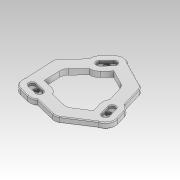
# Autodesk Inventor part: ValveThing2
Saved by Autodesk Inventor 2020 (Build 240168000, 168)
## iProperties
Created: 2022-01-09
Part Number: ValveThing2
Material: Generic
Document SubType Name: Modeling
Designer: DDeGo
Density: 1 g/cm^3
Appearance: Default
Author: DDeGo
Autodesk Inventor part; units mm, degrees
ref_plane "YZ Plane" through (0, 0, 0) normal (1, 0, 0) x (0, 1, 0)
ref_plane "XZ Plane" through (0, 0, 0) normal (0, 1, 0) x (-1, 0, 0)
ref_plane "XY Plane" through (0, 0, 0) normal (0, 0, 1) x (1, 0, 0)
sketch "Block1" plane through (0, 0, 0) normal (0, 0, 1) x (1, 0, 0)
  circle A0 centre (-3.875, 6.7117) radius 2.6
  arc A1 (-0.9902, 6.6954) -> (-5.6639, 8.975) centre (-3.327, 7.8352) ccw
  line L0 (-0.9902, 6.6954) -> (-1.5381, 5.5719)
  line L1 (-6.2119, 7.8515) -> (-5.6639, 8.975)
  line L2 (-1.5381, 5.5719) -> (-2.0861, 4.4484)
  arc A2 (-1.5381, 5.5719) -> (-6.2119, 7.8515) centre (-3.875, 6.7117) ccw
  circle A3 centre (-3.875, 6.7117) radius 1.25
  line L3 (-6.7598, 6.728) -> (-6.2119, 7.8515)
  arc A4 (-6.2119, 7.8515) -> (-1.5381, 5.5719) centre (-3.875, 6.7117) ccw
  arc A5 (-6.7598, 6.728) -> (-2.0861, 4.4484) centre (-4.423, 5.5882) ccw
  line L4 (4.6199, 1.9581) -> (1.25, 6.9542)
  line L5 (1.8, 11.5037) -> (7.107, 3.6357)
  line L6 (-5.3033, -4.2052) -> (-4.0564, -4.118)
  line L7 (-3.6936, -9.3054) -> (-4.9406, -9.3926)
  arc A6 (-4.0564, -4.118) -> (-3.6936, -9.3054) centre (-3.875, -6.7117) ccw
  line L8 (-4.0564, -4.118) -> (-2.8094, -4.0308)
  circle A7 centre (-3.875, -6.7117) radius 1.25
  circle A8 centre (-3.875, -6.7117) radius 2.6
  line L9 (-2.4467, -9.2182) -> (-3.6936, -9.3054)
  arc A9 (-3.6936, -9.3054) -> (-4.0564, -4.118) centre (-3.875, -6.7117) ccw
  arc A10 (-2.4467, -9.2182) -> (-2.8094, -4.0308) centre (-2.628, -6.6245) ccw
  arc A11 (-0.4049, -7.9727) -> (-0.6142, -4.98) centre (-2.628, -6.6245) ccw
  arc A12 (-6.6475, -2.3946) -> (-6.4003, -4.5348) centre (-4.8499, -3.2713) ccw
  line L10 (-4.0057, 3.0219) -> (-6.6475, -2.3946)
  line L11 (-10.8625, -4.193) -> (-6.7021, 4.337)
  arc A13 (-6.7021, 4.337) -> (-4.0057, 3.0219) centre (-4.423, 5.5882) ccw
  arc A14 (9.2065, 2.4902) -> (4.8955, -0.4176) centre (7.051, 1.0363) ccw
  line L12 (5.5945, -1.4539) -> (4.8955, -0.4176)
  line L13 (9.2065, 2.4902) -> (9.9055, 1.4539)
  circle A15 centre (7.75, 0) radius 1.25
  line L14 (9.9055, 1.4539) -> (10.6045, 0.4176)
  arc A16 (9.9055, 1.4539) -> (5.5945, -1.4539) centre (7.75, 0) ccw
  circle A17 centre (7.75, 0) radius 2.6
  arc A18 (5.5945, -1.4539) -> (9.9055, 1.4539) centre (7.75, 0) ccw
  arc A19 (6.2935, -2.4902) -> (10.6045, 0.4176) centre (8.449, -1.0363) ccw
  arc A20 (7.1274, -3.2754) -> (10.8801, -1.9581) centre (8.449, -1.0363) ccw
  line L15 (10.8801, -1.9581) -> (11.3403, -2.6404)
  arc A21 (7.107, 3.6357) -> (4.6199, 1.9581) centre (7.051, 1.0363) ccw
  arc A22 (9.0625, -7.3107) -> (11.3403, -2.6404) centre (8.8532, -4.318) ccw
  arc A23 (5.3975, -4.5596) -> (7.1274, -3.2754) centre (5.258, -2.5645) ccw
  line L16 (9.0625, -7.3107) -> (-0.4049, -7.9727)
  line L17 (-0.6142, -4.98) -> (5.3975, -4.5596)
  line L18 (6.2935, -2.4902) -> (5.5945, -1.4539)
  arc A24 (-5.3033, -4.2052) -> (-4.9406, -9.3926) centre (-5.122, -6.7989) ccw
  arc A25 (-6.4003, -4.5348) -> (-7.1358, -8.4434) centre (-5.122, -6.7989) ccw
  line L19 (-7.1358, -8.4434) -> (-7.9568, -8.5008)
  arc A26 (-10.8625, -4.193) -> (-7.9568, -8.5008) centre (-8.1661, -5.5081) ccw
  arc A27 (-0.7272, 7.8102) -> (-3.7443, 10.4015) centre (-3.327, 7.8352) ccw
  line L20 (-3.7443, 10.4015) -> (-3.3835, 11.1412)
  arc A28 (1.25, 6.9542) -> (-0.7272, 7.8102) centre (-0.4081, 5.8358) ccw
  arc A29 (1.8, 11.5037) -> (-3.3835, 11.1412) centre (-0.6871, 9.8261) ccw
  point P0 (0, 0)
sketch "Block2" plane through (0, 0, 0) normal (0, 0, 1) x (1, 0, 0)
  line L0 (-0.9902, 6.6954) -> (-2.0861, 4.4484)
  arc A0 (-4.0057, 3.0219) -> (-2.0861, 4.4484) centre (-4.423, 5.5882) ccw
  arc A1 (-6.7598, 6.728) -> (-6.7021, 4.337) centre (-4.423, 5.5882) ccw
  circle A2 centre (-3.875, 6.7117) radius 2.1
  line L1 (-6.7598, 6.728) -> (-5.6639, 8.975)
  arc A3 (-2.1873, 10.1721) -> (-5.6639, 8.975) centre (-3.327, 7.8352) ccw
  arc A4 (-0.9902, 6.6954) -> (-0.9193, 6.8539) centre (-3.327, 7.8352) ccw
  line L2 (0.8695, 6.4912) -> (-0.9193, 6.8539)
  line L3 (-2.1873, 10.1721) -> (2.6696, 9.1872)
  arc A5 (2.1301, 5.6494) -> (0.8695, 6.4912) centre (0.472, 4.5311) ccw
  arc A6 (3.9302, 8.3455) -> (2.6696, 9.1872) centre (2.2722, 7.2271) ccw
  line L4 (3.9302, 8.3455) -> (7.107, 3.6357)
  line L5 (4.6199, 1.9581) -> (2.1301, 5.6494)
  line L6 (-0.6142, -4.98) -> (3.8275, -4.6694)
  line L7 (5.2623, -7.5764) -> (-0.4049, -7.9727)
  arc A7 (5.2623, -7.5764) -> (6.6215, -6.9056) centre (5.1228, -5.5813) ccw
  line L8 (9.9029, -3.1918) -> (6.6215, -6.9056)
  arc A8 (9.9029, -3.1918) -> (10.6045, 0.4176) centre (8.449, -1.0363) ccw
  line L9 (9.2065, 2.4902) -> (10.6045, 0.4176)
  arc A9 (9.2065, 2.4902) -> (7.107, 3.6357) centre (7.051, 1.0363) ccw
  arc A10 (4.6199, 1.9581) -> (4.8955, -0.4176) centre (7.051, 1.0363) ccw
  line L10 (6.2935, -2.4902) -> (4.8955, -0.4176)
  arc A11 (6.2935, -2.4902) -> (6.3953, -2.6308) centre (8.449, -1.0363) ccw
  arc A12 (3.8275, -4.6694) -> (5.1868, -3.9986) centre (3.688, -2.6743) ccw
  line L11 (5.1868, -3.9986) -> (6.3953, -2.6308)
  circle A13 centre (7.75, 0) radius 2.1
  line L12 (-7.7156, -6.9803) -> (-9.2912, -2.2816)
  arc A14 (-7.7156, -6.9803) -> (-4.9406, -9.3926) centre (-5.122, -6.7989) ccw
  line L13 (-2.4467, -9.2182) -> (-4.9406, -9.3926)
  arc A15 (-2.4467, -9.2182) -> (-0.4049, -7.9727) centre (-2.628, -6.6245) ccw
  line L14 (-5.3033, -4.2052) -> (-2.8094, -4.0308)
  arc A16 (-5.3033, -4.2052) -> (-5.476, -4.2231) centre (-5.122, -6.7989) ccw
  circle A17 centre (-3.875, -6.7117) radius 2.1
  arc A18 (-0.6142, -4.98) -> (-2.8094, -4.0308) centre (-2.628, -6.6245) ccw
  line L15 (-4.0057, 3.0219) -> (-5.9576, -0.98)
  line L16 (-9.1925, -0.7691) -> (-6.7021, 4.337)
  arc A19 (-5.9576, -0.98) -> (-6.0562, -2.4926) centre (-4.16, -1.8568) ccw
  line L17 (-6.0562, -2.4926) -> (-5.476, -4.2231)
  arc A20 (-9.1925, -0.7691) -> (-9.2912, -2.2816) centre (-7.3949, -1.6458) ccw
  point P0 (0, 0)
  point P1 (0, 0)
sketch "Sketch6" plane through (0, 0, 0) normal (0, 1, 0) x (-1, 0, 0)
  arc A0 (-45, -21.7945) -> (-45, 21.7945) centre (0, 0) ccw
  line L0 (-45, 21.7945) -> (-45, -21.7945)
  dimension "d22" = 50
  dimension "d23" = 45
  constraints: 2 end point, 2 point on circle, 1 centre point, 1 coincident, 1 vertical
  measures "d22" radius of A0
  measures "d23" distance from line of L0 point (0, 0)
extrude "Extrusion6" add sketch "Sketch6" along normal blind 1.4
sketch "Sketch7" plane through (0, 1.4, 0) normal (0, 1, 0) x (1, 0, 0)
  arc A0 (7.5335, 6.4999) -> (6.53, 7.7139) centre (5.6147, 5.9356) ccw projected
  line L0 (0.2576, 10.9422) -> (6.53, 7.7139) projected
  arc A1 (0.2576, 10.9422) -> (-3.4183, 10.8532) centre (-1.5358, 9.0597) ccw projected
  line L1 (-5.1427, 9.0431) -> (-3.4183, 10.8532) projected
  arc A2 (-5.1427, 9.0431) -> (-5.8481, 6.998) centre (-3.2603, 7.2497) ccw projected
  line L2 (-9.3958, 3.2742) -> (-5.8481, 6.998) projected
  arc A3 (-9.3958, 3.2742) -> (-9.9454, 1.7981) centre (-7.9478, 1.8947) ccw projected
  line L3 (-9.605, -5.248) -> (-9.9454, 1.7981) projected
  arc A4 (-9.605, -5.248) -> (-7.69, -8.3869) centre (-7.078, -5.8599) ccw projected
  line L4 (-5.2602, -8.9753) -> (-7.69, -8.3869) projected
  arc A5 (-5.2602, -8.9753) -> (-3.1364, -8.5636) centre (-4.6483, -6.4483) ccw projected
  line L5 (1.8623, -9.7741) -> (-3.1364, -8.5636) projected
  arc A6 (1.8623, -9.7741) -> (3.4155, -9.5121) centre (2.3331, -7.8303) ccw projected
  line L6 (9.3474, -5.6942) -> (3.4155, -9.5121) projected
  arc A7 (9.3474, -5.6942) -> (11.1083, -2.4663) centre (8.6139, -3.1998) ccw projected
  line L7 (10.4029, -0.0678) -> (11.1083, -2.4663) projected
  arc A8 (10.4029, -0.0678) -> (8.9845, 1.5656) centre (7.9086, -0.8013) ccw projected
  line L8 (7.5335, 6.4999) -> (8.9845, 1.5656) projected
  arc A9 (5.7226, 0.6064) -> (5.4142, -1.5349) centre (7.9086, -0.8013) ccw projected
  line L9 (6.0688, -3.761) -> (5.4142, -1.5349) projected
  line L10 (2.8001, -5.8648) -> (6.0688, -3.761) projected
  arc A10 (1.247, -6.1268) -> (2.8001, -5.8648) centre (1.7177, -4.183) ccw projected
  line L11 (-2.3362, -5.2591) -> (1.247, -6.1268) projected
  arc A11 (-2.3362, -5.2591) -> (-4.0363, -3.9214) centre (-4.6483, -6.4483) ccw projected
  line L12 (-6.2915, -3.3753) -> (-4.0363, -3.9214) projected
  line L13 (-6.4791, 0.5074) -> (-6.2915, -3.3753) projected
  arc A12 (-5.9295, 1.9835) -> (-6.4791, 0.5074) centre (-4.4814, 0.6039) ccw projected
  line L14 (-3.3864, 4.6527) -> (-5.9295, 1.9835) projected
  arc A13 (-3.3864, 4.6527) -> (-1.3779, 5.4563) centre (-3.2603, 7.2497) ccw projected
  line L15 (0.2227, 7.1362) -> (-1.3779, 5.4563) projected
  line L16 (3.679, 5.3574) -> (0.2227, 7.1362) projected
  arc A14 (4.6825, 4.1433) -> (3.679, 5.3574) centre (2.7637, 3.5791) ccw projected
  line L17 (5.7226, 0.6064) -> (4.6825, 4.1433) projected
  circle A15 centre (-5.8632, -6.1541) radius 2.1 projected
  circle A16 centre (-2.3981, 8.1547) radius 2.1 projected
  circle A17 centre (8.2612, -2.0006) radius 2.1 projected
  line L18 (45, -21.7945) -> (45, 21.7945) projected
  arc A18 (45, 21.7945) -> (45, -21.7945) centre (0, 0) ccw projected
extrude "Extrusion7" cut sketch "Sketch7" against normal through all contours A9 L9 L10 A10 L11 A11 L12 L13 A12 L14 A13 L15 L16 A14 L17 | A18 L18
sketch "Sketch8" plane through (0, 1.4, 0) normal (0, 1, 0) x (1, 0, 0)
  line L0 (4.6825, 4.1433) -> (5.7226, 0.6064) projected
  arc A0 (5.7226, 0.6064) -> (5.4142, -1.5349) centre (7.9086, -0.8013) ccw projected
  line L1 (5.4142, -1.5349) -> (6.0688, -3.761) projected
  line L2 (6.0688, -3.761) -> (2.8001, -5.8648) projected
  arc A1 (1.247, -6.1268) -> (2.8001, -5.8648) centre (1.7177, -4.183) ccw projected
  line L3 (1.247, -6.1268) -> (-2.3362, -5.2591) projected
  arc A2 (-2.3362, -5.2591) -> (-4.0363, -3.9214) centre (-4.6483, -6.4483) ccw projected
  line L4 (-4.0363, -3.9214) -> (-6.2915, -3.3753) projected
  line L5 (-6.2915, -3.3753) -> (-6.4791, 0.5074) projected
  arc A3 (-5.9295, 1.9835) -> (-6.4791, 0.5074) centre (-4.4814, 0.6039) ccw projected
  line L6 (-5.9295, 1.9835) -> (-3.3864, 4.6527) projected
  arc A4 (-3.3864, 4.6527) -> (-1.3779, 5.4563) centre (-3.2603, 7.2497) ccw projected
  line L7 (-1.3779, 5.4563) -> (0.2227, 7.1362) projected
  line L8 (0.2227, 7.1362) -> (3.679, 5.3574) projected
  arc A5 (4.6825, 4.1433) -> (3.679, 5.3574) centre (2.7637, 3.5791) ccw projected
  line L9 (-3.4183, 10.8532) -> (-5.1427, 9.0431) projected
  arc A6 (-5.1427, 9.0431) -> (-5.8481, 6.998) centre (-3.2603, 7.2497) ccw projected
  line L10 (-5.8481, 6.998) -> (-9.3958, 3.2742) projected
  arc A7 (-9.3958, 3.2742) -> (-9.9454, 1.7981) centre (-7.9478, 1.8947) ccw projected
  line L11 (-9.9454, 1.7981) -> (-9.605, -5.248) projected
  arc A8 (-9.605, -5.248) -> (-7.69, -8.3869) centre (-7.078, -5.8599) ccw projected
  line L12 (-7.69, -8.3869) -> (-5.2602, -8.9753) projected
  arc A9 (-5.2602, -8.9753) -> (-3.1364, -8.5636) centre (-4.6483, -6.4483) ccw projected
  line L13 (-3.1364, -8.5636) -> (1.8623, -9.7741) projected
  arc A10 (1.8623, -9.7741) -> (3.4155, -9.5121) centre (2.3331, -7.8303) ccw projected
  line L14 (3.4155, -9.5121) -> (9.3474, -5.6942) projected
  arc A11 (9.3474, -5.6942) -> (11.1083, -2.4663) centre (8.6139, -3.1998) ccw projected
  line L15 (11.1083, -2.4663) -> (10.4029, -0.0678) projected
  arc A12 (10.4029, -0.0678) -> (8.9845, 1.5656) centre (7.9086, -0.8013) ccw projected
  line L16 (8.9845, 1.5656) -> (7.5335, 6.4999) projected
  arc A13 (7.5335, 6.4999) -> (6.53, 7.7139) centre (5.6147, 5.9356) ccw projected
  line L17 (6.53, 7.7139) -> (0.2576, 10.9422) projected
  arc A14 (0.2576, 10.9422) -> (-3.4183, 10.8532) centre (-1.5358, 9.0597) ccw projected
  arc A15 (-5.0341, 8.9397) -> (-5.6913, 6.9451) centre (-3.2603, 7.2497) ccw
  line L18 (-5.0341, 8.9397) -> (-3.3097, 10.7497)
  arc A16 (0.1695, 10.8188) -> (-3.3097, 10.7497) centre (-1.5358, 9.0597) ccw
  line L19 (0.1695, 10.8188) -> (6.4613, 7.5806)
  arc A17 (7.3896, 6.4576) -> (6.4613, 7.5806) centre (5.6147, 5.9356) ccw
  line L20 (7.3896, 6.4576) -> (8.8603, 1.4562)
  arc A18 (10.259, -0.1101) -> (8.8603, 1.4562) centre (7.9086, -0.8013) ccw
  line L21 (10.259, -0.1101) -> (10.9643, -2.5086)
  arc A19 (9.2846, -5.5562) -> (10.9643, -2.5086) centre (8.6139, -3.1998) ccw
  line L22 (9.2846, -5.5562) -> (3.3343, -9.3859)
  arc A20 (1.8976, -9.6283) -> (3.3343, -9.3859) centre (2.3331, -7.8303) ccw
  line L23 (1.8976, -9.6283) -> (-3.169, -8.4014)
  arc A21 (-5.2249, -8.8295) -> (-3.169, -8.4014) centre (-4.6483, -6.4483) ccw
  line L24 (-5.2249, -8.8295) -> (-7.6547, -8.2411)
  arc A22 (-9.4541, -5.2627) -> (-7.6547, -8.2411) centre (-7.078, -5.8599) ccw
  line L25 (-9.4541, -5.2627) -> (-9.7956, 1.8054)
  arc A23 (-9.2872, 3.1708) -> (-9.7956, 1.8054) centre (-7.9478, 1.8947) ccw
  line L26 (-9.2872, 3.1708) -> (-5.6913, 6.9451)
  line L27 (2.8813, -5.9909) -> (6.2444, -3.8264)
  line L28 (6.2444, -3.8264) -> (5.5581, -1.4926)
  arc A24 (5.8862, 0.5816) -> (5.5581, -1.4926) centre (7.9086, -0.8013) ccw
  line L29 (5.8862, 0.5816) -> (4.8264, 4.1856)
  arc A25 (4.8264, 4.1856) -> (3.7476, 5.4907) centre (2.7637, 3.5791) ccw
  line L30 (3.7476, 5.4907) -> (0.1915, 7.321)
  line L31 (0.1915, 7.321) -> (-1.4865, 5.5597)
  arc A26 (-3.4468, 4.8068) -> (-1.4865, 5.5597) centre (-3.2603, 7.2497) ccw
  line L32 (-3.4468, 4.8068) -> (-6.0381, 2.087)
  arc A27 (-6.0381, 2.087) -> (-6.6289, 0.5002) centre (-4.4814, 0.6039) ccw
  line L33 (-6.6289, 0.5002) -> (-6.4359, -3.4946)
  line L34 (-6.4359, -3.4946) -> (-4.0716, -4.0672)
  arc A28 (-2.4394, -5.3885) -> (-4.0716, -4.0672) centre (-4.6483, -6.4483) ccw
  line L35 (-2.4394, -5.3885) -> (1.2117, -6.2726)
  arc A29 (1.2117, -6.2726) -> (2.8813, -5.9909) centre (1.7177, -4.183) ccw
  point P0 (0, 0)
  dimension "d28" = 0.15
  dimension "d33" = 0.15
  constraints: 36 end point, 30 point on circle, 15 centre point, 31 other
  measures "d28" distance between parallel lines of L10 L26
  measures "d33" distance between parallel lines of L6 L32
extrude "Extrusion8" cut sketch "Sketch8" against normal through all
sketch "Sketch2" plane through (0, 1.4, 1.4) normal (0, 1, 0) x (1, 0, 0)
  line L0 (-4.6483, -5.0483) -> (-7.078, -4.4599) construction
  line L1 (-4.813, -5.7287) -> (-7.2428, -5.1403)
  line L2 (-6.9133, -3.7796) -> (-4.4835, -4.368)
  arc A0 (-4.813, -5.7287) -> (-4.4835, -4.368) centre (-4.6483, -5.0483) ccw
  arc A1 (-6.9133, -3.7796) -> (-7.2428, -5.1403) centre (-7.078, -4.4599) ccw
  line L3 (7.9086, 0.5987) -> (8.6139, -1.7998) construction
  line L4 (7.237, 0.4012) -> (7.9423, -1.9973)
  line L5 (9.2854, -1.6023) -> (8.5801, 0.7961)
  arc A2 (8.5801, 0.7961) -> (7.237, 0.4012) centre (7.9086, 0.5987) ccw
  arc A3 (7.9423, -1.9973) -> (9.2854, -1.6023) centre (8.6139, -1.7998) ccw
  line L6 (-3.2603, 8.6497) -> (-1.5358, 10.4597) construction
  line L7 (-3.7671, 9.1325) -> (-2.0426, 10.9426)
  line L8 (-1.029, 9.9769) -> (-2.7535, 8.1668)
  arc A4 (-3.7671, 9.1325) -> (-2.7535, 8.1668) centre (-3.2603, 8.6497) ccw
  arc A5 (-1.029, 9.9769) -> (-2.0426, 10.9426) centre (-1.5358, 10.4597) ccw
  arc A6 (-5.0341, 10.3397) -> (-5.6913, 8.3451) centre (-3.2603, 8.6497) ccw projected
  arc A7 (0.1695, 12.2188) -> (-3.3097, 12.1497) centre (-1.5358, 10.4597) ccw projected
  arc A8 (9.2846, -4.1562) -> (10.9643, -1.1086) centre (8.6139, -1.7998) ccw projected
  arc A9 (-9.4541, -3.8627) -> (-7.6547, -6.8411) centre (-7.078, -4.4599) ccw projected
  arc A10 (5.8862, 1.9816) -> (5.5581, -0.0926) centre (7.9086, 0.5987) ccw projected
  arc A11 (-3.4468, 6.2068) -> (-1.4865, 6.9597) centre (-3.2603, 8.6497) ccw projected
  arc A12 (-2.4394, -3.9885) -> (-4.0716, -2.6672) centre (-4.6483, -5.0483) ccw projected
  point P0 (0, 0)
  point P1 (-5.8632, -4.7541)
  point P2 (8.2612, -0.6006)
  point P3 (-2.3981, 9.5547)
  dimension "d2" = 0.7
  constraints: 23 end point, 12 point on circle, 12 tangent, 7 concentric, 6 centre point, 3 midpoint, 3 parallel, 2 equal radius, 1 coincident, 1 point on line
  measures "d2" radius of A4
extrude "Extrusion2" cut sketch "Sketch2" against normal blind 0.65
sketch "Sketch3" plane through (0, 0.75, 1.4) normal (0, 1, 0) x (1, 0, 0)
  line L0 (-3.7671, 9.1325) -> (-2.0426, 10.9426) construction
  arc A0 (-3.7671, 9.1325) -> (-2.7535, 8.1668) centre (-3.2603, 8.6497) ccw construction
  line L1 (-1.029, 9.9769) -> (-2.7535, 8.1668) construction
  arc A1 (-1.029, 9.9769) -> (-2.0426, 10.9426) centre (-1.5358, 10.4597) ccw construction
  arc A2 (8.5801, 0.7961) -> (7.237, 0.4012) centre (7.9086, 0.5987) ccw construction
  line L2 (7.9423, -1.9973) -> (7.237, 0.4012) construction
  arc A3 (7.9423, -1.9973) -> (9.2854, -1.6023) centre (8.6139, -1.7998) ccw construction
  line L3 (8.5801, 0.7961) -> (9.2854, -1.6023) construction
  arc A4 (-6.9133, -3.7796) -> (-7.2428, -5.1403) centre (-7.078, -4.4599) ccw construction
  line L4 (-4.813, -5.7287) -> (-7.2428, -5.1403) construction
  arc A5 (-4.813, -5.7287) -> (-4.4835, -4.368) centre (-4.6483, -5.0483) ccw construction
  line L5 (-6.9133, -3.7796) -> (-4.4835, -4.368) construction
  line L6 (-3.2603, 8.6497) -> (-1.5358, 10.4597) construction
  line L7 (7.9086, 0.5987) -> (8.6139, -1.7998) construction
  line L8 (8.5801, 0.7961) -> (9.2854, -1.6023) construction
  line L9 (-4.6483, -5.0483) -> (-7.078, -4.4599) construction
  circle A6 centre (-2.3981, 9.5547) radius 0.7
  circle A7 centre (8.2612, -0.6006) radius 0.7
  circle A8 centre (-5.8632, -4.7541) radius 0.7
  dimension "d32" = 1.4
  constraints: 6 end point, 3 centre point, 3 midpoint, 2 equal radius, 1 parallel
  measures "d32" diameter of A6
extrude "Extrusion3" cut sketch "Sketch3" against normal through all
fillet "Fillet2" radius 0.2 12 edges at (-3.9679, 1.4, 6.6131) (-6.0279, 1.4, 6.8345) (-7.7584, 1.4, 5.6952) (-5.6984, 1.4, 5.4738) (-1.053, 1.4, -9.5665) (-1.8913, 1.4, -7.6719) (-3.7431, 1.4, -6.7429) (-2.9049, 1.4, -8.6376) (7.7111, 1.4, 0.1298) (8.9328, 1.4, 1.8031) (8.8114, 1.4, 3.8714) (7.5897, 1.4, 2.1981)
fillet "Fillet4" radius 0.2 36 edges at (-9.6815, 1.4, -2.5402) (-9.6249, 1.4, 1.7286) (-7.4892, 1.4, -5.0579) (-9.6815, 0, -2.5402) (-9.6249, 0, 1.7286) (-7.4892, 0, -5.0579) (-4.1719, 0, -9.8447) (-1.5845, 0, -11.5092) (-5.5872, 0, -8.0164) (-4.1719, 1.4, -9.8447) (-1.5845, 1.4, -11.5092) (-5.5872, 1.4, -8.0164) (7.0406, 1.4, -7.1143) (8.1249, 1.4, -3.9569) (3.3154, 1.4, -9.1997) (7.0406, 0, -7.1143) (8.1249, 0, -3.9569) (3.3154, 0, -9.1997) (9.736, 1.4, -0.8305) (10.7596, 1.4, 4.3824) (10.6117, 1.4, 1.3094) (10.7596, 0, 4.3824) (9.736, 0, -0.8305) (10.6117, 0, 1.3094) (2.6408, 0, 9.6545) (-0.6357, 0, 9.0148) (6.3095, 0, 7.4711) (2.6408, 1.4, 9.6545) (-0.6357, 1.4, 9.0148) (6.3095, 1.4, 7.4711) (-6.4398, 0, 8.5353) (-9.175, 0, 7.1268) (-4.1488, 0, 8.8469) (-6.4398, 1.4, 8.5353) (-9.175, 1.4, 7.1268) (-4.1488, 1.4, 8.8469)
body "Solid1"
body "Solid2"
